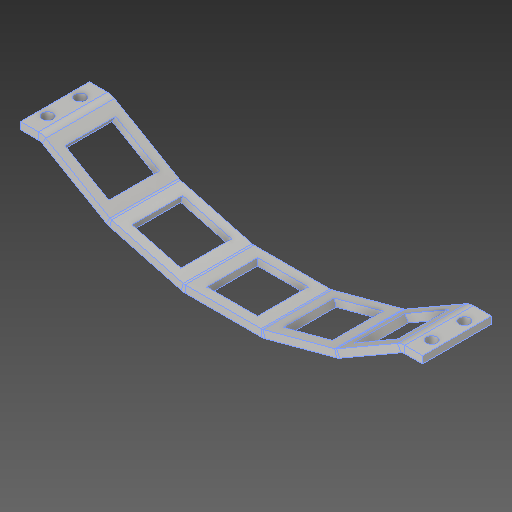
# Autodesk Inventor part: keyplate5
Saved by Autodesk Inventor 2018 (Build 220112000, 112)
## iProperties
Created: 2018-05-25
Part Number: keyplate5
Material: アルミニウム 6061
Document SubType Name: Sheet Metal
Designer: NaMACHAN
Mass: 6.66552 g
Surface Area: 36.5224 cm^2
Volume: 2.46871 cm^3
Density: 2.7 g/cm^3
Flat Pattern Width: 1.9 cm
Flat Pattern Length: 11.7782 cm
Flat Pattern Area: 22.3785 cm^2
Sheet Metal Rule: Al2mm
Sheet Metal Width: 19.000 mm
Sheet Metal Length: 117.782 mm
Sheet Metal Area: 2237.855 mm^2
Appearance: アルミニウム - フラット
Author: NaMACHAN
Autodesk Inventor part; units mm, degrees
ref_plane "YZ Plane" through (0, 0, 0) normal (1, 0, 0) x (0, 1, 0)
ref_plane "XZ Plane" through (0, 0, 0) normal (0, 1, 0) x (-1, 0, 0)
ref_plane "XY Plane" through (0, 0, 0) normal (0, 0, 1) x (1, 0, 0)
sketch "スケッチ1" plane through (0, 0, 0) normal (0, 1, 0) x (-1, 0, 0)
  line L0 (-10.5, -9.5) -> (10.5, -9.5)
  line L1 (10.5, -9.5) -> (10.5, 9.5)
  line L2 (10.5, 9.5) -> (-10.5, 9.5)
  line L3 (-10.5, 9.5) -> (-10.5, -9.5)
  line L4 (-10.5, -9.5) -> (10.5, 9.5) construction
  line L5 (10.5, -9.5) -> (-10.5, 9.5) construction
  line L6 (-7, -7) -> (7, -7)
  line L7 (7, -7) -> (7, 7)
  line L8 (7, 7) -> (-7, 7)
  line L9 (-7, 7) -> (-7, -7)
  line L10 (-7, -7) -> (7, 7) construction
  line L11 (7, -7) -> (-7, 7) construction
  point P0 (0, 0)
  dimension "d0" = 21
  dimension "d1" = 19
  dimension "d2" = 14
  dimension "d3" = 14
  measures "d0" distance of L2.end L1.end
  measures "d1" distance of L1.end L0.end
  measures "d2" distance of L8.end L7.end
  measures "d3" distance of L7.end L6.end
extrude "プレート1" add sketch "スケッチ1" along normal blind 2
sketch "スケッチ2" plane through (-11.0176, 2.0681, 9.5) normal (-0.258819, -0.9659258, 0) x (0.9659258, -0.258819, 0)
  line L0 (0, -19) -> (0, 0)
  line L1 (0, 0) -> (-20.4734, 0)
  line L2 (-20.4734, 0) -> (-20.4734, -19)
  line L3 (-20.4734, -19) -> (0, -19)
  constraints: 6 end point, 1 horizontal, 1 perpendicular, 1 vertical
edge flange "フランジ1" height 21 angle 15 thickness 2 bend radius 2 thickness toward (-0.258819, -0.9659258, 0) relief tear relief width 2 relief depth 1 edges at (-10.5, 2, 0) wall of the first edge with corners at (-11.0176, 2.0681, -9.5) (-11.0176, 2.0681, 9.5) (-30.7934, 7.3671, 9.5) (-30.7934, 7.3671, -9.5)
bend "曲げ1"
corner "コーナー1"
sketch "スケッチ3" plane through (11.0176, 2.0681, -9.5) normal (0.258819, -0.9659258, 0) x (0.9659258, 0.258819, 0)
  line L0 (0, 19) -> (0, 0)
  line L1 (0, 0) -> (20.4734, 0)
  line L2 (20.4734, 0) -> (20.4734, 19)
  line L3 (20.4734, 19) -> (0, 19)
  constraints: 6 end point, 1 horizontal, 1 perpendicular, 1 vertical
edge flange "フランジ2" height 21 angle 15 thickness 2 bend radius 2 thickness toward (0.258819, -0.9659258, 0) relief tear relief width 2 relief depth 1 edges at (10.5, 2, 0) wall of the first edge with corners at (11.0176, 2.0681, 9.5) (11.0176, 2.0681, -9.5) (30.7934, 7.3671, -9.5) (30.7934, 7.3671, 9.5)
bend "曲げ2"
corner "コーナー2"
sketch "スケッチ4" plane through (31.2758, 7.5669, -9.5) normal (0.5, -0.8660254, 0) x (0.8660254, 0.5, 0)
  line L0 (0, 19) -> (0, 0)
  line L1 (0, 0) -> (19.4734, 0)
  line L2 (19.4734, 0) -> (19.4734, 19)
  line L3 (19.4734, 19) -> (0, 19)
  constraints: 8 end point
edge flange "フランジ3" height 20 angle 15 thickness 2 bend radius 2 thickness toward (0.5, -0.8660254, 0) relief tear relief width 2 relief depth 1 edges at (30.7934, 7.3671, 0) wall of the first edge with corners at (31.2758, 7.5669, 9.5) (31.2758, 7.5669, -9.5) (48.1402, 17.3035, -9.5) (48.1402, 17.3035, 9.5)
bend "曲げ3"
corner "コーナー3"
sketch "スケッチ5" plane through (50.1402, 15.8394, -9.5) normal (0, 1, 0) x (1, 0, 0)
  line L0 (0, 19) -> (0, 0)
  line L1 (0, 0) -> (4.9282, 0)
  line L2 (4.9282, 0) -> (4.9282, 19)
  line L3 (4.9282, 19) -> (0, 19)
  constraints: 6 end point, 1 horizontal, 1 perpendicular, 1 vertical
edge flange "フランジ4" height 6 angle 30 thickness 2 bend radius 2 thickness toward (0, 1, 0) relief tear relief width 2 relief depth 1 edges at (48.1402, 17.3035, 0) wall of the first edge with corners at (50.1402, 15.8394, 9.5) (50.1402, 15.8394, -9.5) (55.0684, 15.8394, -9.5) (55.0684, 15.8394, 9.5)
bend "曲げ4"
corner "コーナー4"
sketch "スケッチ32" plane through (-31.2758, 7.5669, 9.5) normal (-0.5, -0.8660254, 0) x (0.8660254, -0.5, 0)
  line L0 (0, -19) -> (0, 0)
  line L1 (0, 0) -> (-20.4734, 0)
  line L2 (-20.4734, 0) -> (-20.4734, -19)
  line L3 (-20.4734, -19) -> (0, -19)
  constraints: 6 end point, 1 horizontal, 1 perpendicular, 1 vertical
edge flange "フランジ12" height 21 angle 15 thickness 2 bend radius 2 thickness toward (-0.5, -0.8660254, 0) relief tear relief width 2 relief depth 1 edges at (-30.7934, 7.3671, 0) wall of the first edge with corners at (-31.2758, 7.5669, -9.5) (-31.2758, 7.5669, 9.5) (-49.0063, 17.8035, 9.5) (-49.0063, 17.8035, -9.5)
bend "曲げ12"
corner "コーナー12"
sketch "スケッチ33" plane through (-11.0176, 2.0681, 9.5) normal (0.258819, 0.9659258, 0) x (0.9659258, -0.258819, 0)
  line L0 (-17.2367, 2.5) -> (-3.2367, 2.5)
  line L1 (-3.2367, 2.5) -> (-3.2367, 16.5)
  line L2 (-3.2367, 16.5) -> (-17.2367, 16.5)
  line L3 (-17.2367, 16.5) -> (-17.2367, 2.5)
  line L4 (-17.2367, 2.5) -> (-3.2367, 16.5) construction
  line L5 (-3.2367, 2.5) -> (-17.2367, 16.5) construction
  line L6 (0.5176, 0) -> (0.5176, 19) projected
  line L7 (-20.4734, 19) -> (0, 19) projected
  point P0 (11.1775, 9.5)
  point P1 (-10.2367, 9.5)
  point P2 (0.5176, 9.5)
  point P3 (-10.2367, 9.5)
  point P4 (-10.2367, 19)
  dimension "d238" = 14
  dimension "d239" = 14
  constraints: 12 end point, 5 midpoint, 2 parallel, 1 horizontal, 1 horizontal alignment, 1 perpendicular, 1 vertical alignment
  measures "d238" distance of L2.end L1.end
  measures "d239" distance of L1.end L0.end
extrude "押し出し14" cut sketch "スケッチ33" against normal blind 10
sketch "スケッチ34" plane through (-49.0063, 17.8035, 9.5) normal (0.5, 0.8660254, 0) x (0.8660254, -0.5, 0)
  line L0 (17.2367, 16.5) -> (3.2367, 16.5)
  line L1 (3.2367, 16.5) -> (3.2367, 2.5)
  line L2 (3.2367, 2.5) -> (17.2367, 2.5)
  line L3 (17.2367, 2.5) -> (17.2367, 16.5)
  line L4 (17.2367, 16.5) -> (3.2367, 2.5) construction
  line L5 (3.2367, 16.5) -> (17.2367, 2.5) construction
  line L6 (20.991, 19) -> (20.991, 0) projected
  line L7 (0, 19) -> (20.4734, 19) projected
  point P0 (51.3424, 9.5)
  point P1 (10.2367, 9.5)
  point P2 (10.2367, 9.5)
  point P3 (20.991, 9.5)
  point P4 (10.2367, 9.5)
  point P5 (10.2367, 19)
  dimension "d242" = 14
  dimension "d243" = 14
  constraints: 12 end point, 6 midpoint, 2 parallel, 1 horizontal, 1 horizontal alignment, 1 perpendicular, 1 vertical alignment
  measures "d242" distance of L2.end L1.end
  measures "d243" distance of L1.end L0.end
extrude "押し出し15" cut sketch "スケッチ34" against normal blind 10
sketch "スケッチ35" plane through (11.0176, 2.0681, 9.5) normal (-0.258819, 0.9659258, 0) x (0.9659258, 0.258819, 0)
  line L0 (17.2367, 16.5) -> (3.2367, 16.5)
  line L1 (3.2367, 16.5) -> (3.2367, 2.5)
  line L2 (3.2367, 2.5) -> (17.2367, 2.5)
  line L3 (17.2367, 2.5) -> (17.2367, 16.5)
  line L4 (17.2367, 16.5) -> (3.2367, 2.5) construction
  line L5 (3.2367, 16.5) -> (17.2367, 2.5) construction
  line L6 (20.4734, 19) -> (0, 19) projected
  line L7 (0, 19) -> (0, 0) projected
  point P0 (-11.1775, 9.5)
  point P1 (10.2367, 9.5)
  point P2 (10.2367, 9.5)
  point P3 (10.2367, 19)
  point P4 (10.2367, 9.5)
  point P5 (0, 9.5)
  dimension "d246" = 14
  dimension "d247" = 14
  constraints: 12 end point, 6 midpoint, 2 parallel, 1 horizontal, 1 horizontal alignment, 1 perpendicular, 1 vertical alignment
  measures "d246" distance of L2.end L1.end
  measures "d247" distance of L1.end L0.end
extrude "押し出し16" cut sketch "スケッチ35" against normal blind 10
sketch "スケッチ36" plane through (31.2758, 7.5669, 9.5) normal (-0.5, 0.8660254, 0) x (0.8660254, 0.5, 0)
  line L0 (16.7367, 16.5) -> (2.7367, 16.5)
  line L1 (2.7367, 16.5) -> (2.7367, 2.5)
  line L2 (2.7367, 2.5) -> (16.7367, 2.5)
  line L3 (16.7367, 2.5) -> (16.7367, 16.5)
  line L4 (16.7367, 16.5) -> (2.7367, 2.5) construction
  line L5 (2.7367, 16.5) -> (16.7367, 2.5) construction
  line L6 (-0.5176, 0) -> (-0.5176, 19) projected
  line L7 (19.4734, 19) -> (0, 19) projected
  point P0 (-30.869, 9.5)
  point P1 (9.7367, 9.5)
  point P2 (9.7367, 9.5)
  point P3 (-0.5176, 9.5)
  point P4 (9.7367, 19)
  dimension "d250" = 14
  dimension "d251" = 14
  constraints: 12 end point, 5 midpoint, 2 parallel, 1 horizontal, 1 horizontal alignment, 1 perpendicular, 1 vertical alignment
  measures "d250" distance of L2.end L1.end
  measures "d251" distance of L1.end L0.end
extrude "押し出し17" cut sketch "スケッチ36" against normal blind 10
sketch "スケッチ37" plane through (-51.0063, 16.3394, -9.5) normal (0, 1, 0) x (-1, 0, 0)
  line L0 (0, 19) -> (0, 0)
  line L1 (0, 0) -> (4.9282, 0)
  line L2 (4.9282, 0) -> (4.9282, 19)
  line L3 (4.9282, 19) -> (0, 19)
  constraints: 6 end point, 1 horizontal, 1 perpendicular, 1 vertical
edge flange "フランジ13" height 6 angle 30 thickness 2 bend radius 2 thickness toward (0, 1, 0) relief tear relief width 2 relief depth 1 edges at (-50.0063, 16.0715, 0) wall of the first edge with corners at (-51.0063, 16.3394, 9.5) (-51.0063, 16.3394, -9.5) (-55.9345, 16.3394, -9.5) (-55.9345, 16.3394, 9.5)
bend "曲げ13"
corner "コーナー13"
sketch "スケッチ40" plane through (-55.9345, 18.3394, 9.5) normal (0, 1, 0) x (1, 0, 0)
  line L0 (106.0747, 19) -> (111.0029, 19) projected
  line L1 (106.0747, 0) -> (111.0029, 0) projected
  line L2 (0, 19) -> (4.9282, 19) projected
  point P0 (55.9345, 9.5)
  point P1 (108.5388, 14)
  point P2 (108.5388, 5)
  point P3 (2.4641, 14)
  point P4 (2.4641, 5)
  point P5 (108.5388, 19)
  point P6 (2.4641, 19)
  dimension "d282" = 5
  dimension "d283" = 5
  constraints: 4 vertical alignment, 2 horizontal alignment, 2 midpoint
  measures "d282" distance from line of L0 point (108.539, 14)
  measures "d283" distance from line of L1 point (108.539, 5)
hole "穴8" at (52.6043, 18.3394, -4.5) at (52.6043, 18.3394, 4.5) at (-53.4704, 18.3394, -4.5) at (-53.4704, 18.3394, 4.5) direction (0, -1, 0) diameter 3 end through all
equation "\"d4\" = Thickness"
equation "\"d5\" = BendReliefWidth"
equation "\"d6\" = BendReliefDepth"
equation "\"d7\" = MinimumRemnant"
equation "\"d8\" = TransitionRadius"
equation "\"d11\" = BendRadius"
equation "\"d12\" = CornerReliefSize"
equation "\"d13\" = GapSize"
equation "\"d14\" = JacobiRadiusSize"
equation "\"d15\" = BendReliefWidth"
equation "\"d16\" = BendReliefDepth"
equation "\"d17\" = MinimumRemnant"
equation "\"d18\" = TransitionRadius"
equation "\"d21\" = BendRadius"
equation "\"d22\" = CornerReliefSize"
equation "\"d23\" = GapSize"
equation "\"d24\" = JacobiRadiusSize"
equation "\"d25\" = BendReliefWidth"
equation "\"d26\" = BendReliefDepth"
equation "\"d27\" = MinimumRemnant"
equation "\"d28\" = TransitionRadius"
equation "\"d31\" = BendRadius"
equation "\"d32\" = CornerReliefSize"
equation "\"d33\" = GapSize"
equation "\"d34\" = JacobiRadiusSize"
equation "\"d35\" = BendReliefWidth"
equation "\"d36\" = BendReliefDepth"
equation "\"d37\" = MinimumRemnant"
equation "\"d38\" = TransitionRadius"
equation "\"d41\" = BendRadius"
equation "\"d42\" = CornerReliefSize"
equation "\"d43\" = GapSize"
equation "\"d44\" = JacobiRadiusSize"
equation "\"BendRadius\" = Thickness"
equation "\"BendReliefWidth\" = Thickness"
equation "\"BendReliefDepth\" = 0.5 * Thickness"
equation "\"CornerReliefSize\" = 4 * Thickness"
equation "\"MinimumRemnant\" = 2 * Thickness"
equation "\"TransitionRadius\" = BendRadius"
equation "\"JacobiRadiusSize\" = BendRadius"
equation "\"GapSize\" = Thickness"
equation "\"Thickness\" = 2"
